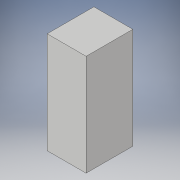
# Autodesk Inventor part: petite-batterie
Saved by Autodesk Inventor 2019 (Build 230136000, 136)
## iProperties
Created: 2019-03-31
Part Number: petite-batterie
Material: Generic
Document SubType Name: Modeling
Designer: franc
Density: 1 g/cm^3
Appearance: Default
Author: franc
Autodesk Inventor part; units mm, degrees
ref_plane "YZ Plane" through (0, 0, 0) normal (1, 0, 0) x (0, 1, 0)
ref_plane "XZ Plane" through (0, 0, 0) normal (0, 1, 0) x (-1, 0, 0)
ref_plane "XY Plane" through (0, 0, 0) normal (0, 0, 1) x (1, 0, 0)
sketch "Esquisse1" plane through (0, 0, 0) normal (0, 1, 0) x (-1, 0, 0)
  line L0 (29.2373, 27.2034) -> (-20.7627, 27.2034)
  line L1 (-20.7627, 27.2034) -> (-20.7627, -32.7966)
  line L2 (-20.7627, -32.7966) -> (29.2373, -32.7966)
  line L3 (29.2373, -32.7966) -> (29.2373, 27.2034)
  point P0 (0, 0)
  dimension "d0" = 60
  dimension "d1" = 50
  constraints: 8 end point, 2 parallel, 1 horizontal, 1 perpendicular
  measures "d0" distance of L2.end L0.start
  measures "d1" distance of L1.end L2.end
extrude "Extrusion1" add sketch "Esquisse1" along normal blind 130
